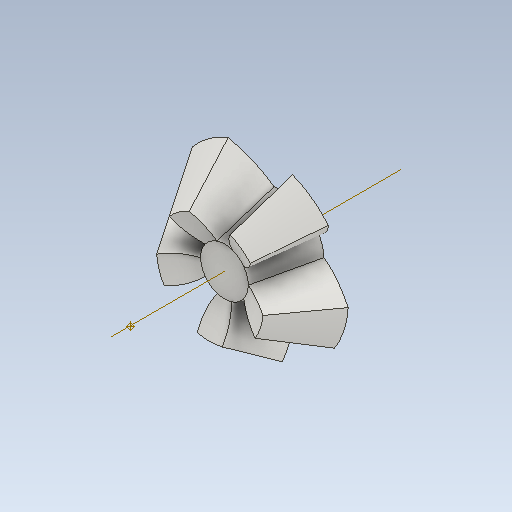
# Autodesk Inventor part: Bevel Gear2
Saved by Autodesk Inventor 2020.2 (Build 242310000, 310)
## iProperties
CustomPartVersion: 1
Created: 2020-02-28
Part Number: Bevel Gear2
Material: Steel, Mild
Document SubType Name: Modeling
Designer: deli
Categories: <?xml version="1.0" encoding="UTF-16"?> <MemberInstance><Categories><FamilyTemplate><FamilyTemplateParameter ValueType="xs:double" Id="1" ObjectReferenceKey="da_z" ObjectType="kUserParameterObject"/><FamilyTemplateParameter ValueType="xs:double" Id="2" ObjectReferenceKey="da_b" ObjectType="kUserParameterObject"/><FamilyTemplateParameter ValueType="xs:double" Id="3" ObjectReferenceKey="da_beta" ObjectType="kUserParameterObject"/><FamilyTemplateParameter ValueType="xs:double" Id="4" ObjectReferenceKey="da_dae" ObjectType="kUserParameterObject"/><FamilyTemplateParameter ValueType="xs:double" Id="5" ObjectReferenceKey="da_ve" ObjectType="kUserParameterObject"/><FamilyTemplateParameter ValueType="xs:double" Id="6" ObjectReferenceKey="da_omega" ObjectType="kUserParameterObject"/><FamilyTemplateParameter ValueType="xs:string" Id="7" ObjectReferenceKey="EAIAABAAAAAAHwAAAAAAAIAAAAAAAAAA" ObjectType="83914240" SubObjectId="SurfaceGeometry"/></FamilyTemplate><ParamToTemplateMap><ParamToTemplate CategoryParameter="//CategoryParameter[@InternalName='046C89C9-8512-4d59-83FE-43B91F4F132A']" TemplateParameter="1"/><ParamToTemplate CategoryParameter="//CategoryParameter[@InternalName='2552DF32-E462-4b46-AEBF-C6C7768E72AC']" TemplateParameter="2"/><ParamToTemplate CategoryParameter="//CategoryParameter[@InternalName='C9EE641D-15FC-4fae-A226-E94C4372FDD7']" TemplateParameter="3"/><ParamToTemplate><ParamToTemplate CategoryParameter="//CategoryParameter[@InternalName='00B6519A-459B-49c7-AD84-2E56D39A5744']" ConstantValue="-0.000000"/></ParamToTemplate><ParamToTemplate><ParamToTemplate CategoryParameter="//CategoryParameter[@InternalName='04B31F0E-C7A6-4894-AA32-9629BEFACF47']" ConstantValue="1.000000"/></ParamToTemplate><ParamToTemplate><ParamToTemplate CategoryParameter="//CategoryParameter[@InternalName='43CBEC2E-7847-49e7-A936-2F7889FCB2D9']" ConstantValue="0.200000"/></ParamToTemplate><ParamToTemplate><ParamToTemplate CategoryParameter="//CategoryParameter[@InternalName='B1EFC894-105D-4ebd-86BF-FA20ED196853']" ConstantValue="0.300000"/></ParamToTemplate><ParamToTemplate><ParamToTemplate CategoryParameter="//CategoryParameter[@InternalName='51175063-3D10-4879-93E8-6246FE8B403D']" ConstantValue="2061532430.657340"/></ParamToTemplate><ParamToTemplate><ParamToTemplate CategoryParameter="//CategoryParameter[@InternalName='A3A52E27-4454-46a9-B0BD-C932399B70AF']" ConstantValue="0.300000"/></ParamToTemplate><ParamToTemplate CategoryParameter="//CategoryParameter[@InternalName='2A200944-5A8C-41ca-B96E-8520D2E510F1']" TemplateParameter="4"/><ParamToTemplate><ParamToTemplate CategoryParameter="//CategoryParameter[@InternalName='1A637F62-92C8-44bc-B81F-10802510B579']" ConstantValue="0.981497"/></ParamToTemplate><ParamToTemplate CategoryParameter="//CategoryParameter[@InternalName='B52DD4BE-6863-48fb-BF58-89EF6F9EC65C']" TemplateParameter="5"/><ParamToTemplate><ParamToTemplate CategoryParameter="//CategoryParameter[@InternalName='3956BFF2-84D2-457d-93C2-9B0613DEBA67']" ConstantValue="0.716027"/></ParamToTemplate><ParamToTemplate CategoryParameter="//CategoryParameter[@InternalName='739CFA02-461B-4bf8-8049-181FCAD8B28F']" TemplateParameter="6"/><ParamToTemplate><ParamToTemplate CategoryParameter="//CategoryParameter[@InternalName='A27E999F-E2CE-4481-8A2A-EBF499C4C3C5']" ConstantValue="-0.000000"/></ParamToTemplate><ParamToTemplate><ParamToTemplate CategoryParameter="//CategoryParameter[@InternalName='9E1B4470-B2D3-4ff1-B813-535BB4CDF51A']" ConstantValue="3523220.976809"/></ParamToTemplate><ParamToTemplate><ParamToTemplate CategoryParameter="//CategoryParameter[@InternalName='F8452263-BFF6-458c-9FB1-07C4B99E95CD']" ConstantValue="11397033.805607"/></ParamToTemplate><ParamToTemplate><ParamToTemplate CategoryParameter="//CategoryParameter[@InternalName='3E3BB259-FD49-497f-8171-6EBC954A3479']" ConstantValue="2.000000"/></ParamToTemplate><ParamToTemplate CategoryParameter="//CategoryParameter[@InternalName='27C3BAF2-7550-4e4b-AE2C-0DB134B7D9B7']" TemplateParameter="7"/></ParamToTemplateMap><Category DisplayName="Gear" InternalName="DC85795E-93AB-48d5-8EEE-5A27447B64BD" Mnemonic="Gear"><CategoryParameter DisplayName="z" InternalName="046C89C9-8512-4d59-83FE-43B91F4F132A" Mnemonic="z"/><CategoryParameter DisplayName="b" InternalName="2552DF32-E462-4b46-AEBF-C6C7768E72AC" Mnemonic="b"/><CategoryParameter DisplayName="||b|" InternalName="C9EE641D-15FC-4fae-A226-E94C4372FDD7" Mnemonic="beta"/><CategoryParameter DisplayName="x" InternalName="00B6519A-459B-49c7-AD84-2E56D39A5744" Mnemonic="x"/><CategoryParameter DisplayName="a*" InternalName="04B31F0E-C7A6-4894-AA32-9629BEFACF47" Mnemonic="a"/><CategoryParameter DisplayName="c*" InternalName="43CBEC2E-7847-49e7-A936-2F7889FCB2D9" Mnemonic="c"/><CategoryParameter DisplayName="r|.f|*" InternalName="B1EFC894-105D-4ebd-86BF-FA20ED196853" Mnemonic="rf"/><CategoryParameter DisplayName="E" InternalName="51175063-3D10-4879-93E8-6246FE8B403D" Mnemonic="E"/><CategoryParameter DisplayName="||m|" InternalName="A3A52E27-4454-46a9-B0BD-C932399B70AF" Mnemonic="mi"/><Category DisplayName="BevelGear" InternalName="0C98F69A-0C2B-4791-B2FE-7691BB227E77" Mnemonic="BevelGear"><CategoryParameter DisplayName="d|.ae|" InternalName="2A200944-5A8C-41ca-B96E-8520D2E510F1" Mnemonic="dae"/><CategoryParameter DisplayName="d|.ai|" InternalName="1A637F62-92C8-44bc-B81F-10802510B579" Mnemonic="dai"/><CategoryParameter DisplayName="A|.e|" InternalName="B52DD4BE-6863-48fb-BF58-89EF6F9EC65C" Mnemonic="ve"/><CategoryParameter DisplayName="A|.i|" InternalName="3956BFF2-84D2-457d-93C2-9B0613DEBA67" Mnemonic="vi"/><CategoryParameter DisplayName="||S|" InternalName="739CFA02-461B-4bf8-8049-181FCAD8B28F" Mnemonic="omega"/><CategoryParameter DisplayName="x|.t|" InternalName="A27E999F-E2CE-4481-8A2A-EBF499C4C3C5" Mnemonic="xt"/><CategoryParameter DisplayName="||s||.Flim|" InternalName="9E1B4470-B2D3-4ff1-B813-535BB4CDF51A" Mnemonic="sFlim"/><CategoryParameter DisplayName="||s||.Hlim|" InternalName="F8452263-BFF6-458c-9FB1-07C4B99E95CD" Mnemonic="sHlim"/><CategoryParameter DisplayName="type" InternalName="3E3BB259-FD49-497f-8171-6EBC954A3479" Mnemonic="type"/><CategoryParameter DisplayName="PitchDiameter" InternalName="27C3BAF2-7550-4e4b-AE2C-0DB134B7D9B7" Mnemonic="IDS_PITCHDIAM"/></Category></Category></Categories></MemberInstance>
Mass: 60.9118 g
Surface Area: 34.3074 cm^2
Volume: 7.7496 cm^3
Density: 7.86 g/cm^3
Appearance: Steel
d48: 0.0000 in
d49: 0.0000 in
d50: 90.00 deg
d52: 0.0000 in
d53: 0.0000 in
d54: 0.00 deg
Author: deli
Autodesk Inventor part; units mm, degrees
ref_plane "Mesh Plane2" through (0, 0, 0) normal (0.809017, 0.5877853, 0) x (0, 0, 1)
sketch "Teeth Body Sketch" plane through (0, 0, 0) normal (1, 0, 0) x (0, 1, 0)
  line L0 (0, 0) -> (3.623786, -14.063107) construction
  line L1 (3.623786, -14.063107) -> (8.103418, -11.823291)
  line L2 (8.103418, -11.823291) -> (0, 0) construction
  line L3 (6.35, -12.7) -> (0, 0) construction
  line L4 (2.19459, -8.516715) -> (4.907486, -7.160267)
  line L5 (3.623786, -14.063107) -> (2.19459, -8.516715)
  line L6 (8.103418, -11.823291) -> (4.907486, -7.160267)
  line L7 (0, -39.386751) -> (0, 6.564458)
  line L8 (0, -12.7) -> (8.103418, -12.7) construction
  dimension "d0" = 12.7
  dimension "d1" = 7.24757
  dimension "d2" = 16.20684
  dimension "d3" = 5.6
  dimension "d4" = 11.82329
  constraints: 16 end point, 4 point on line, 3 perpendicular, 2 collinear, 1 horizontal alignment, 1 vertical alignment
  measures "d0" diameter of L3.start L7
  measures "d1" diameter of L0.end L7
  measures "d2" diameter of L1.end L7
  measures "d3" distance between parallel lines of L1 L4
  measures "d4" vertical distance of L1.end L0.start
revolve "Teeth Body" add sketch "Teeth Body Sketch" angle 360 about axis through (0, 0, 0) along (0, 0, 1)
ref_plane "Tooth Plane" through (0, 6.35, -12.7) normal (0, -0.4472136, 0.8944272) x (1, 0, 0)
sketch "Start Sketch" plane through (0, 6.35, -12.7) normal (0, -0.4472136, 0.8944272) x (1, 0, 0)
  line L0 (0, -23.505131) -> (0, 10.644758)
  arc A0 (-0.938283, -3.645557) -> (-7.75304, 4.501286) centre (-10.066138, -4.357259) ccw
  arc A1 (7.75304, 4.501286) -> (0.938283, -3.645557) centre (10.066138, -4.357259) ccw
  line L1 (-0.938283, -3.645557) -> (0.938283, -3.645557)
  arc A2 (7.75304, 4.501286) -> (-7.75304, 4.501286) centre (0, -18.626575) ccw
  point P0 (0, -7.099516)
  dimension "d7" = 2.29951
  dimension "d8" = 3.87249
  dimension "d9" = 5.53129
  dimension "d57" = 10.56241
  dimension "d58" = 3.45051
  constraints: 6 point on circle, 3 centre point, 3 symmetric about line, 2 end point, 1 perpendicular, 1 vertical alignment, 1 other
sketch "End Sketch" plane through (0, 3.733613, -7.467226) normal (0, -0.4472136, 0.8944272) x (1, 0, 0)
  line L0 (0, -15.35404) -> (0, 6.953444)
  arc A0 (-0.612908, -2.381315) -> (-5.064462, 2.940388) centre (-6.57543, -2.846215) ccw
  arc A1 (5.064462, 2.940388) -> (0.612908, -2.381315) centre (6.57543, -2.846215) ccw
  line L1 (-0.612908, -2.381315) -> (0.612908, -2.381315)
  arc A2 (5.064462, 2.940388) -> (-5.064462, 2.940388) centre (0, -12.167256) ccw
  point P0 (0, -4.174306)
  dimension "d12" = 1.35204
  dimension "d15" = 2.27691
  dimension "d16" = 3.25223
  dimension "d59" = 6.21039
  dimension "d60" = 2.0288
  constraints: 6 point on circle, 3 centre point, 3 symmetric about line, 2 end point, 1 vertical alignment, 1 other
loft "Loft" cut profiles "Start Sketch", "End Sketch"
pattern_circular "Circular Pattern" count 5 over 360 about axis through (0, 0, 0) along (0, 0, 1) of "Loft"
ref_plane "End Plane" through (0, 3.733613, -7.467226) normal (0, -0.4472136, 0.8944272) x (1, 0, 0)
sketch3d "3D Sketch Right"
ref_plane "End Plane Right" through (-1.514593, 3.412605, -7.467226) normal (0.1814185, -0.4087632, 0.8944272) x (0.9140223, 0.405664, 0)
sketch "End Sketch Right" plane through (-1.514593, 3.412605, -7.467226) normal (0.1814185, -0.4087632, 0.8944272) x (0.9140223, 0.405664, 0)
  arc A0 (-0.612908, -2.381321) -> (-5.064462, 2.940383) centre (-6.57543, -2.84622) ccw
  line L0 (0, -21.459956) -> (0, 13.059349)
  arc A1 (5.064462, 2.940383) -> (0.612908, -2.381321) centre (6.57543, -2.84622) ccw
  line L1 (-0.612908, -2.381321) -> (0.612908, -2.381321)
  arc A2 (5.064462, 2.940383) -> (-5.064462, 2.940383) centre (0, -12.167262) ccw
  point P0 (0, -4.174306)
  dimension "d70" = 2.27691
  dimension "d71" = 3.25223
  dimension "d72" = 1.35204
  dimension "d73" = 2.0288
  dimension "d74" = 6.21039
  constraints: 6 point on circle, 3 centre point, 3 symmetric about line, 2 end point, 1 perpendicular, 1 vertical alignment, 1 other
feature "Loft Right" [suppressed]
pattern_circular "Circular Pattern Right" [suppressed]
sketch3d "3D Sketch Left"
ref_plane "End Plane Left" through (1.470704, 3.412605, -7.454722) normal (-0.1765642, -0.4096977, 0.8949709) x (0.9183482, -0.3957733, 0)
sketch "End Sketch Left" plane through (1.470704, 3.412605, -7.454722) normal (-0.1765642, -0.4096977, 0.8949709) x (0.9183482, -0.3957733, 0)
  line L0 (0, -37.67995) -> (0, 20.657227)
  arc A0 (-0.612908, -2.379015) -> (-5.064462, 2.942689) centre (-6.57543, -2.843914) ccw
  arc A1 (5.064462, 2.942689) -> (0.612908, -2.379015) centre (6.57543, -2.843914) ccw
  line L1 (-0.612908, -2.379015) -> (0.612908, -2.379015)
  ellipse E0 centre (0, -3.194371) end of major axis (4.907486, -3.194371) minor radius 4.392057
  arc A2 (5.064462, 2.942689) -> (-5.064462, 2.942689) centre (0, -12.164956) ccw
  point P0 (0, -4.164141)
  dimension "d56" = 4.39206
  dimension "d30" = 1.35204
  dimension "d31" = 2.27691
  dimension "d32" = 3.25223
  dimension "d61" = 6.21039
  dimension "d62" = 2.0288
  constraints: 6 point on circle, 3 centre point, 3 symmetric about line, 2 end point, 1 vertical alignment, 2 other
feature "Loft Left" [suppressed]
pattern_circular "Circular Pattern Left" [suppressed]
sketch "Body Sketch" plane through (0, 0, 0) normal (1, 0, 0) x (0, 1, 0)
  line L0 (0, -35.037536) -> (0, -19.530831)
  line L1 (3.623786, -14.063107) -> (2.19459, -8.516715)
  line L2 (2.19459, -8.516715) -> (0, -8.516715)
  line L3 (3.623786, -14.063107) -> (0, -14.063107)
  constraints: 4 end point, 2 perpendicular, 2 point on line
sketch "Body Sketch outline for Fix Body" plane through (0, 0, 0) normal (1, 0, 0) x (0, 1, 0)
  line L0 (0, -14.063107) -> (3.623786, -14.063107)
  line L1 (0, -8.516715) -> (0, -14.063107)
  line L2 (2.19459, -8.516715) -> (0, -8.516715)
  line L3 (3.623786, -14.063107) -> (2.19459, -8.516715)
revolve "Fix Body" add sketch "Body Sketch outline for Fix Body" angle 360 about axis through (0, 0, 0) along (0, 0, 1)
sketch "Sketch6" plane through (0, 0, 0) normal (1, 0, 0) x (0, 1, 0)
  line L0 (6.35, -12.7) -> (0, 0)
  line L1 (0, -37.799919) -> (0, 6.299986)
surface revolve "Pitch Diameter" sketch "Sketch6" angle 360 about axis through (0, 0, 0) along (0, 0, 1) shown no curves L0
equation "\"d0\" = da_de"
equation "\"d1\" = da_dfe"
equation "\"d2\" = da_dae"
equation "\"d3\" = da_b"
equation "\"d4\" = da_ve"
equation "\"d7\" = fd_rr"
equation "\"d8\" = fd_x"
equation "\"d9\" = fd_y"
equation "\"d57\" = 0.5 * fd_dva + 0.3 * da_he"
equation "\"d58\" = 0.5 * fd_dva - 1.12 * da_he"
equation "\"da_teethtype\" = 0"
equation "\"da_b\" = 5.6"
equation "\"da_de\" = 12.7"
equation "\"da_dae\" = 16.20684"
equation "\"da_dfe\" = 7.24757"
equation "\"da_le\" = 14.19903"
equation "\"da_omega\" = 90deg"
equation "\"da_beta\" = 0"
equation "\"da_delta\" = 26.565051deg"
equation "\"da_alpha\" = 20deg"
equation "\"da_he\" = 5.00838"
equation "\"da_ve\" = 11.82329"
equation "\"da_zv\" = 5.59017"
equation "\"fd_loft\" = da_b + 0.05 * da_he"
equation "\"fd_x\" = fd_x1 + fd_x2"
equation "\"fd_y\" = fd_y1 - fd_y2"
equation "\"fd_dd\" = fd_dva - 0.8 * da_he"
equation "\"da_dvw\" = 14.19903"
equation "\"d11\" = fd_loft"
equation "\"da_dm\" = 10.1956"
equation "\"da_x\" = 0"
equation "\"da_m\" = 2.54"
equation "\"d50\" = da_omega"
equation "\"fd_rr\" = 2.299508"
equation "\"fd_dva\" = 18.119793"
equation "\"fd_x1\" = 1.968763"
equation "\"fd_x2\" = 1.903728"
equation "\"fd_y1\" = 6.821077"
equation "\"fd_y2\" = 1.289789"
body "Solid1"
body "Srf1"
